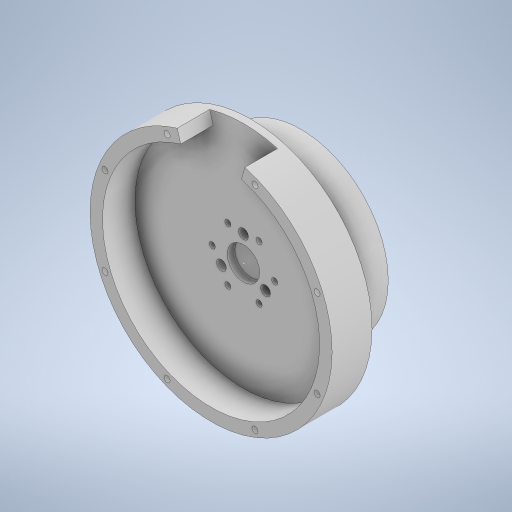
# Autodesk Inventor part: legparts_01(five)
Saved by Autodesk Inventor 2024.3 (Build 283343000, 343)
## iProperties
Created: 2024-10-20
Part Number: legparts_01(five)
Material: 一般
Document SubType Name: Modeling
Designer: 佐藤智貴
Density: 1 g/cm^3
Appearance: 既定
Author: 佐藤智貴
Autodesk Inventor part; units mm, degrees
ref_plane "YZ Plane" through (0, 0, 0) normal (1, 0, 0) x (0, 1, 0)
ref_plane "XZ Plane" through (0, 0, 0) normal (0, 1, 0) x (-1, 0, 0)
ref_plane "XY Plane" through (0, 0, 0) normal (0, 0, 1) x (1, 0, 0)
sketch "スケッチ1" plane through (0, 0, 0) normal (0, 0, 1) x (1, 0, 0)
  circle A0 centre (0, 0) radius 48.5
  dimension "d0" = 97
  constraints: 1 centre point, 1 coincident
  measures "d0" diameter of A0
extrude "押し出し1" add sketch "スケッチ1" along normal blind 24
sketch "スケッチ2" plane through (0, 0, 24) normal (0, 0, 1) x (1, 0, 0)
  line L0 (0, 0) -> (-27.4547, 66.2816)
  line L1 (0, 0) -> (26.2443, 63.3594)
  circle A0 centre (0, 0) radius 46
  line L2 (0, 0) -> (0, 57.2216)
  point P0 (-17.6034, 42.4985)
  point P1 (17.6034, 42.4985)
  point P2 (-42.4985, -17.6034)
  point P3 (-42.4985, 17.6034)
  point P4 (17.6034, -42.4985)
  point P5 (-17.6034, -42.4985)
  point P6 (42.4985, 17.6034)
  point P7 (42.4985, -17.6034)
  dimension "d3" = 92
  dimension "d4" = 45
  dimension "d8" = 360
  dimension "d45" = 22.5
  constraints: 6 end point, 2 point on circle, 2 point on line, 1 centre point, 1 coincident, 1 vertical, 9 other
  measures "d3" diameter of A0
  measures "d4" angle of L1 L0
  measures "d45" angle of L0 L2
hole "穴1" at (-17.6034, 42.4985, 24) at (17.6034, 42.4985, 24) at (-42.4985, -17.6034, 24) at (-42.4985, 17.6034, 24) at (17.6034, -42.4985, 24) at (-17.6034, -42.4985, 24) at (42.4985, 17.6034, 24) at (42.4985, -17.6034, 24) direction (0, 0, -1) diameter 2.459 end through all
sketch "スケッチ3" plane through (0, 0, 0) normal (0, 0, -1) x (-1, 0, 0)
  circle A0 centre (0, 0) radius 12.5
  line L0 (0, 0) -> (-8.9989, 15.5865)
  line L1 (0, 0) -> (0, 21.1985)
  point P0 (-6.25, 10.8253)
  point P1 (-12.5, 0)
  point P2 (-6.25, -10.8253)
  point P3 (6.25, -10.8253)
  point P4 (12.5, 0)
  point P5 (6.25, 10.8253)
  dimension "d17" = 25
  dimension "d18" = 30
  dimension "d21" = 360
  constraints: 4 end point, 1 coincident, 1 point on line, 1 vertical, 10 other
  measures "d18" angle of L1 L0
hole "穴2" at (6.25, 10.8253, 0) at (12.5, 0, 0) at (6.25, -10.8253, 0) at (-6.25, -10.8253, 0) at (-12.5, 0, 0) at (-6.25, 10.8253, 0) direction (0, 0, 1) diameter 2.459 end through all
sketch "スケッチ4" plane through (0, 0, 0) normal (0, 0, -1) x (-1, 0, 0)
  circle A0 centre (0, 0) radius 10.2
  point P0 (0, 10.2)
  point P1 (0, 10.2)
  point P2 (-8.8335, -5.1)
  point P3 (8.8335, -5.1)
  dimension "d30" = 20.4
  dimension "d33" = 360
  constraints: 2 coincident, 1 vertical alignment, 6 other
hole "穴3" at (0, 10.2, 0) at (8.8335, -5.1, 0) at (-8.8335, -5.1, 0) direction (0, 0, 1) diameter 4 end through all
sketch "スケッチ5" plane through (0, 0, 24) normal (0, 0, 1) x (1, 0, 0)
  circle A0 centre (0, 0) radius 43.5
  dimension "d42" = 87
  constraints: 1 centre point, 1 coincident
  measures "d42" diameter of A0
extrude "押し出し2" cut sketch "スケッチ5" against normal blind 21
sketch "スケッチ6" plane through (0, 0, 24) normal (0, 0, 1) x (1, 0, 0)
  circle A0 centre (0, 0) radius 48.5 projected
  circle A1 centre (0, 0) radius 43.5 projected
  line L0 (-13.5797, 46.5601) -> (0, 0)
  line L1 (0, 0) -> (13.6731, 46.8801)
  circle A2 centre (-17.6034, 42.4985) radius 1.2295 projected
  circle A3 centre (17.6034, 42.4985) radius 1.2295 projected
  arc A4 (13.5797, 46.5601) -> (-13.5797, 46.5601) centre (0, 0) ccw
  arc A5 (12.1798, 41.7601) -> (-12.1798, 41.7601) centre (0, 0) ccw
  dimension "d46" = 5
  dimension "d47" = 5
  constraints: 8 point on circle, 4 end point, 3 point on line, 2 centre point, 2 concentric
  measures "d46" distance from line of L0 A2.centre
  measures "d47" distance from line of L1 A3.centre
extrude "押し出し3" cut sketch "スケッチ6" against normal blind 21 contours L1 A1 L0 A0 picked at (-1.3696, 46.624)
sketch "スケッチ7" plane through (0, 0, 0) normal (0, 0, -1) x (-1, 0, 0)
  circle A0 centre (0, 0) radius 6.5
  dimension "d50" = 13
  constraints: 1 centre point, 1 coincident
  measures "d50" diameter of A0
extrude "押し出し4" cut sketch "スケッチ7" against normal blind 10
sketch "スケッチ8" plane through (0, 0, 24) normal (0, 0, 1) x (1, 0, 0)
  circle A0 centre (0, 0) radius 48.5
  constraints: 1 centre point, 1 coincident
extrude "押し出し5" cut sketch "スケッチ8" against normal blind 8
sketch "スケッチ9" plane through (0, 0, 0) normal (0, 0, -1) x (-1, 0, 0)
  circle A0 centre (0, 0) radius 35
  dimension "d55" = 70
  constraints: 1 centre point, 1 coincident
  measures "d55" diameter of A0
extrude "押し出し6" add sketch "スケッチ9" along normal blind 20
sketch "スケッチ10" plane through (0, 0, 3) normal (0, 0, 1) x (1, 0, 0)
  point P0 (0, 0)
